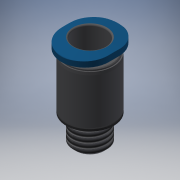
# Autodesk Inventor part: fc17-135
Saved by Autodesk Inventor 2017.1 (Build 211199000, 199)
## iProperties
Category: Pneumatics
Company: Autodesk Inc.
Created: 2016-12-21
Part Number: fc17-135
Catalog Web Link: https://www.festo.com/net/en-ca_ca/SupportPortal/default.aspx?tab=0&q=183740
Description: QSM-I-U-M (USA)-Push-in fitting
Vendor: AndyMark Inc.
Document SubType Name: Modeling
Designer: Autodesk Inc.
Manufacturer: FESTO
Mass: 4 g
Surface Area: 10.5719 cm^2
Volume: 0.736602 cm^3
Density: 1 g/cm^3
Material: Generic
Appearance: PSOLRGB-175-175-175
Title: 183740 QSM-M7-1/4-I-U-M
Author: Autodesk Inc.
Comments: Push-in fitting
Keywords: FIRST Choice
Autodesk Inventor part; units mm, degrees
sketch "Sketch_1" plane through (0, 0, 0) normal (1, 0, 0) x (0, 1, 0)
  line L0 (0, -5.5) -> (0, 13.4)
  line L1 (0, 13.4) -> (3.4785, 13.4)
  line L2 (3.4785, 13.4) -> (5.7347, 13.0022)
  arc A0 (5.9, 12.8052) -> (5.7347, 13.0022) centre (5.7, 12.8052) ccw
  line L3 (5.9, 12.8052) -> (5.9, 11.9)
  line L4 (5.9, 11.9) -> (4.2535, 11.9)
  arc A1 (4.2535, 11.9) -> (3.8785, 11.525) centre (4.2535, 11.525) ccw
  line L5 (3.8785, 11.525) -> (3.8785, 11)
  line L6 (3.8785, 11) -> (4.5136, 11)
  line L7 (4.5136, 11) -> (4.655, 10.8586)
  line L8 (4.655, 10.8586) -> (4.655, 10.6)
  line L9 (4.655, 10.6) -> (4.858, 10.6)
  line L10 (4.858, 10.6) -> (4.9, 10)
  line L11 (4.9, 10) -> (4.9, 0.6)
  line L12 (4.9, 0.6) -> (4.8, 0.5)
  line L13 (4.8, 0.5) -> (4.9, 0.4)
  line L14 (4.9, 0.4) -> (4.9, 0)
  line L15 (4.9, 0) -> (3.5, 0)
  line L16 (3.5, 0) -> (3.5, -4.8865)
  line L17 (3.5, -4.8865) -> (2.8865, -5.5)
  line L18 (2.8865, -5.5) -> (0, -5.5)
  line L19 (0, -5.5) -> (0, 13.4)
  constraints: 40 end point, 4 point on circle, 2 centre point
revolve "Revolution1" add sketch "Sketch_1" angle 360 about axis through (0, 0, -5.5) along (0, 0, -1)
thread "Thread1" size "M7x1" class "6g" standard "ISO Metric profile" length 4.3865
sketch "Sketch_2" plane through (0, 0, 13.4) normal (0, 0, 1) x (1, 0, 0)
  line L0 (-11.8, -11.8) -> (11.8, -11.8)
  line L1 (11.8, -11.8) -> (11.8, 11.8)
  line L2 (11.8, 11.8) -> (-11.8, 11.8)
  line L3 (-11.8, 11.8) -> (-11.8, -11.8)
  line L4 (-4.9, 1) -> (-4.9, -1)
  arc A0 (-4.9, -1) -> (4.9, -1) centre (0, -1) ccw
  line L5 (4.9, -1) -> (4.9, 1)
  arc A1 (4.9, 1) -> (-4.9, 1) centre (0, 1) ccw
  constraints: 12 end point, 4 point on circle, 2 centre point
extrude "Extrusion1" cut sketch "Sketch_2" against normal blind 1.5
sketch "Sketch_3" plane through (0, 0, -5.5) normal (0, 0, 1) x (1, 0, 0)
  line L0 (-2, -1.1547) -> (0, -2.3094)
  line L1 (0, -2.3094) -> (2, -1.1547)
  line L2 (2, -1.1547) -> (2, 1.1547)
  line L3 (2, 1.1547) -> (0, 2.3094)
  line L4 (0, 2.3094) -> (-2, 1.1547)
  line L5 (-2, 1.1547) -> (-2, -1.1547)
  constraints: 12 end point
extrude "Extrusion2" cut sketch "Sketch_3" along normal blind 7.2
sketch "Sketch_4" plane through (0, 0, 0) normal (1, 0, 0) x (0, 1, 0)
  line L0 (0, 1.7) -> (0, 13.4)
  line L1 (0, 13.4) -> (3.4785, 13.4)
  arc A0 (3.4785, 13.4) -> (3.1785, 13.1) centre (3.4785, 13.1) ccw
  line L2 (3.1785, 13.1) -> (3.1785, 1.7)
  line L3 (3.1785, 1.7) -> (0, 1.7)
  line L4 (0, 1.7) -> (0, 13.4)
  constraints: 10 end point, 2 point on circle, 1 centre point
revolve "Revolution2" cut sketch "Sketch_4" angle 360 about axis through (0, 0, 1.7) along (0, 0, -1)
ref_plane "ANBAU_XY" through (0, 0, 0) normal (0, 0, -1) x (1, 0, 0)
ref_plane "ANBAU_YZ" through (0, 0, 0) normal (1, 0, 0) x (0, -1, 0)
ref_plane "ANBAU_ZX" through (0, 0, 0) normal (0, -1, 0) x (0, 0, -1)
ref_plane "ANBAU_STD_XY" through (0, 0, 0) normal (0, 0, 1) x (1, 0, 0)
ref_plane "ANBAU_STD_YZ" through (0, 0, 0) normal (1, 0, 0) x (0, 1, 0)
ref_plane "ANBAU_STD_ZX" through (0, 0, 0) normal (0, 1, 0) x (0, 0, 1)
ref_plane "CPV_XY" through (0, 0, 0) normal (0, 0, 1) x (1, 0, 0)
ref_plane "CPV_YZ" through (0, 0, 0) normal (1, 0, 0) x (0, 1, 0)
ref_plane "CPV_ZX" through (0, 0, 0) normal (0, 1, 0) x (0, 0, 1)
ref_plane "CPV_ANBAU_XY" through (0, 0, 0) normal (0, 0, 1) x (1, 0, 0)
ref_plane "CPV_ANBAU_YZ" through (0, 0, 0) normal (1, 0, 0) x (0, 1, 0)
ref_plane "CPV_ANBAU_ZX" through (0, 0, 0) normal (0, 1, 0) x (0, 0, 1)
body "Solid1"
